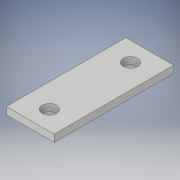
# Autodesk Inventor part: montageplatte_rad_vorne
Saved by Autodesk Inventor 2019 (Build 230136000, 136)
## iProperties
Created: 2021-05-30
Part Number: montageplatte_rad_vorne
Material: Generisch
Document SubType Name: Modeling
Designer: Lukas
Density: 1 g/cm^3
Appearance: Vorgabe
Author: Lukas
Autodesk Inventor part; units mm, degrees
ref_plane "YZ Plane" through (0, 0, 0) normal (1, 0, 0) x (0, 1, 0)
ref_plane "XZ Plane" through (0, 0, 0) normal (0, 1, 0) x (-1, 0, 0)
ref_plane "XY Plane" through (0, 0, 0) normal (0, 0, 1) x (1, 0, 0)
sketch "Skizze1" plane through (0, 0, 0) normal (0, 1, 0) x (-1, 0, 0)
  line L0 (0, 0) -> (-10, 0)
  line L1 (-10, 0) -> (-10, -25)
  line L2 (-10, -25) -> (0, -25)
  line L3 (0, -25) -> (0, 0)
  dimension "d0" = 10
  dimension "d1" = 25
  constraints: 8 end point, 2 parallel, 1 coincident, 1 horizontal, 1 perpendicular
  measures "d0" distance of L0.start L0.end
  measures "d1" distance of L2.end L0.start
extrude "Extrusion1" add sketch "Skizze1" along normal blind 1.5
sketch "Skizze2" plane through (0, 1.5, 0) normal (0, 1, 0) x (1, 0, 0)
  line L0 (0, 0) -> (10, 0) projected
  line L1 (10, 0) -> (10, 25) projected
  point P0 (5, 4)
  point P1 (5, 21)
  dimension "d4" = 17
  dimension "d6" = 4
  dimension "d7" = 5
  dimension "d8" = 5
  measures "d4" distance of point (5, 21) point (5, 4)
  measures "d6" distance from line of L0 point (5, 4)
  measures "d7" distance from line of L1 point (5, 4)
  measures "d8" distance from line of L1 point (5, 21)
hole "Bohrung1" at (5, 1.5, -4) at (5, 1.5, -21) direction (0, -1, 0) diameter 3 end through all
